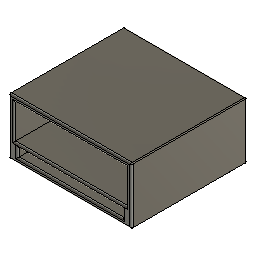
adruino3.31 exterior (Autodesk Fusion 360 design; units mm, degrees)
Autodesk Fusion 360 part; units mm, degrees
sketch "Sketch1" plane through (0, 0, 0) normal (0, 0, 1) x (1, 0, 0)
  line L0 (-25, 25) -> (35, 25)
  line L1 (35, 25) -> (35, -27)
  line L2 (35, -27) -> (-25, -27)
  line L3 (-25, -27) -> (-25, 25)
  dimension "d1" = 60
  dimension "d2" = 52
  constraint perpendicular L0 L1
  constraint parallel L0 L2
  constraint parallel L1 L3
  constraint horizontal L0
  measures "d1" distance of L0.start L0.end
  measures "d2" distance of L0.start L2.end
extrude "Extrude1" add sketch "Sketch1" along normal blind 35
extrude "Extrude2" add 1 faces at (-5, 25, 11.6667) along direction (0, 1, 0) blind 5
extrude "Extrude3" add 1 faces at (15, -27, 11.6667) along direction (0, -1, 0) blind 3
extrude "Extrude4" add 1 faces at (35, 10, 11.6667) along direction (1, 0, 0) blind 15
sketch "Sketch2" plane through (0, 30, 0) normal (0, 1, 0) x (-1, 0, 0)
  line L0 (-50, 0) -> (25, 0)
  line L1 (25, 0) -> (25, 35)
  line L2 (25, 35) -> (-50, 35)
  line L3 (-50, 35) -> (-50, 0)
  line L4 (-45, 30) -> (-45, -21)
  line L5 (-45, -21) -> (20, -21)
  line L6 (20, -21) -> (20, 30)
  line L7 (20, 30) -> (-45, 30)
  dimension "d11" = 51
  dimension "d12" = 65
  constraint perpendicular L4 L5
  constraint parallel L4 L6
  constraint parallel L5 L7
  constraint perpendicular L2 L4
  measures "d11" distance of L4.start L4.end
  measures "d12" distance of L4.start L6.end
extrude "Extrude5" add 1 faces at (0, -10, 0) along direction (0, 0, -1) blind 30
extrude "Extrude6" cut sketch "Sketch2" against normal blind 59 contours L0 L4 L6 L7
extrude "Extrude7" cut 1 faces at (23.3333, 10.3333, 0) along direction (0, 0, -1) blind 25
extrude "Extrude8" add 1 faces at (0, -10, -30) along direction (0, 0, -1) blind 6
extrude "Extrude9" cut 1 faces at (50, -10, 11.3333) along direction (-1, 0, 0) blind 2
extrude "Extrude10" cut 1 faces at (-25, 10, -12.3333) along direction (1, 0, 0) blind 2
extrude "Extrude11" cut 1 faces at (0.6667, 10, 35) along direction (0, 0, -1) blind 2
extrude "Extrude12" cut 1 faces at (0.6667, -10, -36) along direction (0, 0, 1) blind 3
sketch "Sketch6" plane through (0, 0, 0) normal (0, 1, 0) x (1, 0, 0)
  line L0 (43, 25) -> (43, 28)
  line L1 (45, 28) -> (-20, 28)
  line L2 (-20, 28) -> (-20, 30)
  line L3 (-20, 30) -> (45, 30)
  line L4 (45, 30) -> (45, 28)
  line L5 (30, 30) -> (30, 33)
  dimension "d31" = 3
  constraint vertical L0
  constraint perpendicular L1 L2
  constraint parallel L1 L3
  constraint parallel L2 L4
  constraint perpendicular L0 L1
  constraint coincident L3 L5.start
  constraint perpendicular L3 L5
  measures "d31" distance of L0.start L0.end
extrude "Extrude13" cut sketch "Sketch6" along normal blind 30 and the other way blind 38
extrude "Extrude14" add 1 faces at (23.3333, -29, 11.6667) along direction (0, 1, 0) blind 2
sketch "Sketch7" plane through (0, 0, 0) normal (0, 1, 0) x (1, 0, 0)
sketch "Sketch8" plane through (0, 0, 0) normal (0, 1, 0) x (1, 0, 0)
  line L0 (45, 5) -> (-20, 5)
  line L1 (-20, 5) -> (-20, 25)
  line L2 (-20, 25) -> (45, 25)
  line L3 (45, 25) -> (45, 5)
  constraint horizontal L0
  constraint vertical L1
  constraint horizontal L2
  constraint vertical L3
extrude "Extrude15" cut sketch "Sketch8" against normal blind 68
extrude "Extrude16" add 1 faces at (1.6667, 11, 30) along direction (0, 0, -1) blind 10
extrude "Extrude17" cut 1 faces at (0.6667, 10, 33) along direction (0, 0, -1) blind 10
extrude "Extrude18" add 1 faces at (1.6667, 11, 20) along direction (0, 0, -1) blind 0.5
extrude "Extrude19" cut 1 faces at (0.6667, 10, 23) along direction (0, 0, -1) blind 0.5
extrude "Extrude20" add 1 faces at (1.6667, 11, 19.5) along direction (0, 0, -1) blind 1.5
extrude "Extrude21" cut 1 faces at (0.6667, 10, 22.5) along direction (0, 0, -1) blind 0.5
sketch "Sketch9" plane through (0, 0, 0) normal (0, 1, 0) x (1, 0, 0)
extrude "Extrude22" cut 1 faces at (0.6667, 10, 22) along direction (0, 0, -1) blind 1
extrude "Extrude23" add 1 faces at (1.6667, 11, 18) along direction (0, 0, -1) blind 3
extrude "Extrude24" cut 1 faces at (0.6667, 10, 21) along direction (0, 0, -1) blind 3
sketch "Sketch10" plane through (0, 0, 0) normal (0, 1, 0) x (1, 0, 0)
extrude "Extrude25" add 1 faces at (23.3333, -29, -5) along direction (0, 0, -1) blind 8
extrude "Extrude26" add 1 faces at (-22, 30, -13.3333) along direction (0, 1, 0) blind 5
sketch "Sketch11" plane through (0, 35, 0) normal (0, 1, 0) x (-1, 0, 0)
  line L0 (23, 18) -> (-48, 18)
  line L1 (-48, 18) -> (-48, -33)
  line L2 (-48, -33) -> (23, -33)
  line L3 (23, -33) -> (23, 18)
  line L4 (-45, -30) -> (-45, -28)
  line L5 (-45, -28) -> (20, -28)
  line L6 (20, -28) -> (20, -30)
  line L7 (20, -30) -> (-45, -30)
  line L8 (-45, -25) -> (-45, 15)
  line L9 (-45, 15) -> (20, 15)
  line L10 (20, 15) -> (20, -25)
  line L11 (20, -25) -> (-45, -25)
extrude "Extrude27" add sketch "Sketch11" along normal blind 2
extrude "Extrude28" cut 1 faces at (23.3333, -29, -13) along direction (0, 0, 1) blind 5
extrude "Extrude29" cut 1 faces at (23.3333, -29, -8) along direction (0, 0, 1) blind 3
extrude "Extrude30" add 1 faces at (23.3333, -5.6667, 15) along direction (0, 0, -1) blind 15
extrude "Extrude31" cut 1 faces at (24.3333, 14.6667, 18) along direction (0, 0, -1) blind 15
extrude "Extrude32" add 1 faces at (23.3333, -5.6667, 0) along direction (0, 0, -1) blind 5
extrude "Extrude33" cut 1 faces at (24.3333, 14.6667, 3) along direction (0, 0, -1) blind 5
extrude "Extrude34" add 1 faces at (45, 14.6667, -28.6667) along direction (-1, 0, 0) blind 2
extrude "Extrude35" add 1 faces at (-20, -7.6667, -28.6667) along direction (1, 0, 0) blind 2
extrude "Extrude36" cut 1 faces at (22.6667, -7.6667, -28) along direction (0, 0, 1) blind 1
extrude "Extrude37" cut 1 faces at (2.3333, -7.6667, -30) along direction (0, 0, -1) blind 1
extrude "Extrude38" cut 1 faces at (2.3333, -7.6667, -31) along direction (0, 0, -1) blind 1
extrude "Extrude39" add 1 faces at (24.3333, -7.6667, -33) along direction (0, 0, -1) blind 1
extrude "Extrude40" add 1 faces at (24.3333, -7.6667, -34) along direction (0, 0, -1) blind 1
fillet "Fillet1" radius 1 1 faces at (-20.3333, 37, -30.6667)
fillet "Fillet2" radius 1 1 faces at (-20.3333, -30, -30.6667)
fillet "Fillet4" radius 0.5 3 edges at (47.7071, 36.7071, -2.2929) (48, 3.5, -2) (47.7071, -29.7071, -2.2929)
fillet "Fillet5" radius 0.5 3 edges at (47.7071, 36.7071, -34.7071) (48, 3.5, -35) (47.7071, -29.7071, -34.7071)
fillet "Fillet6" radius 0.5 3 edges at (-22.7071, -29.7071, -2.2929) (-23, 3.5, -2) (-22.7071, 36.7071, -2.2929)
fillet "Fillet7" radius 0.5 3 edges at (-22.7071, -29.7071, -34.7071) (-23, 3.5, -35) (-22.7071, 36.7071, -34.7071)
